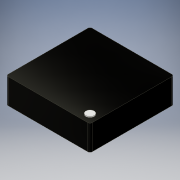
# Autodesk Inventor part: VICOR_PI3546
Saved by Autodesk Inventor 2019.4 (Build 234330000, 330)
## iProperties
Created: 2019-12-30
Part Number: VICOR_PI3546
Material: Generic
Document SubType Name: Modeling
Designer: Jorian Bruslind
Density: 1 g/cm^3
Appearance: Gunmetal
Author: Jorian Bruslind
Autodesk Inventor part; units mm, degrees
ref_plane "YZ Plane" through (0, 0, 0) normal (1, 0, 0) x (0, 1, 0)
ref_plane "XZ Plane" through (0, 0, 0) normal (0, 1, 0) x (-1, 0, 0)
ref_plane "XY Plane" through (0, 0, 0) normal (0, 0, 1) x (1, 0, 0)
sketch "Sketch1" plane through (0, 0, 0) normal (0, 1, 0) x (-1, 0, 0)
  line L0 (0, 0) -> (10, 0)
  line L1 (10, 0) -> (10, -10)
  line L2 (10, -10) -> (0, -10)
  line L3 (0, -10) -> (0, 0)
  dimension "d0" = 10
  dimension "d1" = 10
  constraints: 8 end point, 2 parallel, 1 horizontal, 1 perpendicular
  measures "d0" distance of L1.end L2.end
  measures "d1" distance of L0.end L1.end
extrude "Extrusion1" add sketch "Sketch1" along normal blind 3
fillet "Fillet1" radius 0.25 4 edges at (0, 1.5, 0) (0, 1.5, -10) (-10, 1.5, 0) (-10, 1.5, -10)
sketch "Sketch2" plane through (0, 3, 0) normal (0, 1, 0) x (1, 0, 0)
  line L0 (0, 0) -> (0, 1)
  line L1 (0, 1) -> (-1, 1)
  circle A0 centre (-1, 1) radius 0.5
  dimension "d5" = 1
  dimension "d6" = 1
  dimension "d7" = 1
  constraints: 4 end point, 1 centre point, 1 coincident, 1 perpendicular, 1 vertical
  measures "d5" distance of L0.start L0.end
  measures "d6" distance of L0.end L1.end
  measures "d7" diameter of A0
extrude "Extrusion2" add sketch "Sketch2" along normal blind 0.1
sketch "Sketch3" plane through (0, 0, 0) normal (0, -1, 0) x (1, 0, 0)
  line L0 (-0.25, 0) -> (-9.75, 0) projected
  line L1 (0, -9.75) -> (0, -0.25) projected
  line L2 (-0.25, -0.8) -> (-0.8, -0.8)
  line L3 (-0.8, -0.8) -> (-0.8, -0.25)
  line L4 (-0.8, -0.25) -> (-0.25, -0.25)
  line L5 (-0.25, -0.25) -> (-0.25, -0.8)
  line L6 (-0.25, -0.8) -> (-0.8, -0.25) construction
  line L7 (-0.8, -0.8) -> (-0.25, -0.25) construction
  point P0 (-0.525, -0.525)
  dimension "d16" = 0.55
  dimension "d17" = 0.55
  dimension "d18" = 0.25
  dimension "d19" = 0.8
  constraints: 12 end point, 2 midpoint, 2 parallel, 1 horizontal, 1 perpendicular
  measures "d16" distance of L3.end L4.end
  measures "d17" distance of L2.end L3.end
  measures "d18" distance between parallel lines of L1 L5
  measures "d19" distance between parallel lines of L0 L2
extrude "Extrusion3" add sketch "Sketch3" along normal blind 0.1
pattern_linear "Rectangular Pattern1" count 10 spacing 1 along (0, 0, -1) count 10 spacing 1 along (-1, 0, 0) of "Extrusion3"
body "Solid1"
